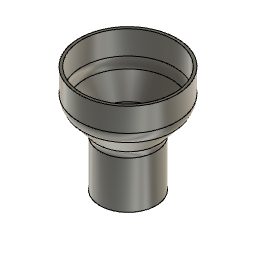
Soap Drainer v2 (Autodesk Fusion 360 design; units mm, degrees)
Autodesk Fusion 360 part; units mm, degrees
sketch "Sketch1" plane through (0, 0, 0) normal (0, 0, 1) x (1, 0, 0) in component "funnel"
  circle A0 centre (0, 0) radius 17.75
  dimension "d1" = 35.5
  constraint coincident A0.centre origin
  measures "d1" diameter of A0
extrude "Extrude2" add sketch "Sketch1" along normal blind 11 in component "funnel"
ref_plane "WorkPlane1" through (0, 0, -10) normal (0, 0, 1) x (1, 0, 0) in component "funnel"
sketch "Sketch2" plane through (0, 0, -10) normal (0, 0, 1) x (1, 0, 0) in component "funnel"
  circle A0 centre (0, 0) radius 8.75
  circle A1 centre (0, 0) radius 9.75
  circle A2 centre (0, 0) radius 17.75
  dimension "d7" = 1
  dimension "d10" = 9
  measures "d7" distance of A0 A1
  measures "d10" distance of A0 A2
loft "Loft1" add profiles "Sketch1", "Sketch2" section 1 section 2 contours A0 | A1 in component "funnel"
extrude "Extrude3" add 1 faces at (1.6592, 0.958, -10) along direction (0, 0, -1) blind 20 in component "funnel"
fillet "Fillet1" radius 5.5 2 edges at (-9.0902, -3.5258, -10) (-16.5488, -6.4187, 0) in component "funnel"
shell "Shell1" thickness 1 outward yes removed faces 2 at (2.6955, 3.38, 11) at (1.6592, 0.958, -30) in component "funnel"
component "funnel" placed x (1, 0, 0) y (0, 1, 0) z (0, 0, 1) at (0, 0, 0)
